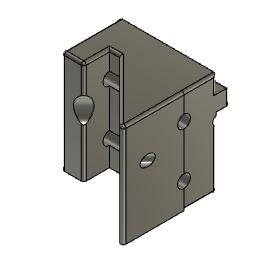
porte miroir ok v3 (Autodesk Fusion 360 design; units mm, degrees)
Autodesk Fusion 360 part; units mm, degrees
sketch "Sketch1" plane through (0, 0, 0) normal (0, 0, 1) x (1, 0, 0)
  line L0 (0, 0) -> (-12.5, 0)
  line L1 (-12.5, 0) -> (-12.5, -10)
  line L2 (0, 0) -> (25, -25)
  line L3 (0, 0) -> (25, 0)
  line L4 (25, 0) -> (25, -25)
  line L5 (-12.5, 0) -> (24.9893, 0)
  line L6 (24.9893, 0) -> (24.9893, 12.5)
  line L7 (24.9893, 12.5) -> (-12.5, 12.5)
  line L8 (-12.5, 12.5) -> (-12.5, 0)
  line L9 (-4, 0) -> (-4, -10)
  line L10 (-12.5, -10) -> (-4, -10)
  dimension "d27" = 12.5
  dimension "d28" = 12.5
  dimension "d29" = 10
  constraint coincident L0.start L2.start
  constraint horizontal L0
  constraint vertical L1
  constraint horizontal L5
  constraint vertical L6
  constraint horizontal L7
  constraint vertical L8
  constraint coincident L5 L9.start
  constraint perpendicular L9 L10
  measures "d27" distance of L0.start L0.end
  measures "d28" distance of L0.end L7.end
  measures "d29" distance of L0.end L1.end
extrude "Extrude7" add sketch "Sketch1" along normal blind 40
sketch "Sketch9" plane through (-12.5, 0, 0) normal (-1, 0, 0) x (0, -1, 0)
  line L0 (-12.5, 0) -> (10, 0)
  line L1 (10, 0) -> (10, 40)
  line L2 (10, 40) -> (-12.5, 40)
  line L3 (-12.5, 40) -> (-12.5, 0)
  circle A0 centre (0, 30) radius 2.5
  circle A1 centre (0, 10) radius 2.5
  dimension "d32" = 5
  dimension "d33" = 5
  dimension "d34" = 10
  dimension "d35" = 10
  dimension "d36" = 20
  measures "d32" diameter of A0
  measures "d33" diameter of A1
  measures "d34" distance of L2 A0.centre
  measures "d35" distance of L0 A1.centre
  measures "d36" distance of A0.centre A1.centre
extrude "Extrude8" cut sketch "Sketch9" against normal blind 50 contours A0 | A1
sketch "Sketch10" plane through (0, 0, 0) normal (-0.707107, -0.707107, 0) x (0.707107, -0.707107, 0)
  line L0 (0, 27.5) -> (0, 12.5)
  ellipse E0 centre (0, 10) end of major axis (3.5355, 10) minor radius 2.5 (0, 7.5) -> (0, 12.5) ccw
  line L1 (0, 7.5) -> (0, 0)
  line L2 (0, 0) -> (35.3553, 0)
  line L3 (35.3553, 0) -> (35.3553, 40)
  line L4 (35.3553, 40) -> (0, 40)
  line L5 (0, 40) -> (0, 32.5)
  ellipse E1 centre (0, 30) end of major axis (3.5355, 30) minor radius 2.5 (0, 27.5) -> (0, 32.5) ccw
  line L6 (17.6777, 24) -> (27.6777, 24)
  circle A0 centre (7.6777, 24) radius 2.1
  circle A1 centre (27.6777, 24) radius 2.1
  dimension "d41" = 4.2
  dimension "d42" = 4.2
  constraint coincident L6.end A1.centre
  measures "d41" diameter of A0
  measures "d42" diameter of A1
extrude "Extrude9" cut sketch "Sketch10" against normal blind 50 contours A0 | A1
sketch "Sketch11" plane through (0, 12.5, 0) normal (0, 1, 0) x (-1, 0, 0)
  ellipse E0 centre (-23.3579, 24) end of major axis (-26.3277, 24) minor radius 2.1 (-24.9893, 22.2452) -> (-24.9893, 25.7548) ccw
  line L0 (-24.9893, 22.2452) -> (-24.9893, 0)
  line L1 (-24.9893, 0) -> (12.5, 0)
  line L2 (12.5, 0) -> (12.5, 40)
  line L3 (12.5, 40) -> (-24.9893, 40)
  line L4 (-24.9893, 40) -> (-24.9893, 25.7548)
  circle A0 centre (-12.5453, 29.9363) radius 2.05
  dimension "d45" = 4.1
  measures "d45" diameter of A0
extrude "Extrude10" cut sketch "Sketch11" against normal blind 50 contours A0
ref_plane "WorkPlane1" through (6.2446, 7.5, 20) normal (0, 1, 0) x (-1, 0, 0)
sketch "Sketch12" plane through (6.2446, 7.5, 20) normal (0, 1, 0) x (1, 0, 0)
  circle A0 centre (6.3004, -9.9317) radius 4.1
  dimension "d49" = 8.2
  measures "d49" diameter of A0
extrude "Extrude11" cut sketch "Sketch12" against normal blind 50
move_face "OffsetFaces2" offset -2 1 faces at (11.1129, 7.5, 26.8414)
sketch "Sketch13" plane through (0, 12.5, 0) normal (0, 1, 0) x (-1, 0, 0)
  circle A0 centre (-12.5453, 29.9363) radius 2.05
  ellipse E0 centre (-23.3579, 24) end of major axis (-26.3277, 24) minor radius 2.1 (-24.9893, 22.2452) -> (-24.9893, 25.7548) ccw
  line L0 (-24.9893, 22.2452) -> (-24.9893, 0)
  line L1 (-24.9893, 0) -> (12.5, 0)
  line L2 (12.5, 0) -> (12.5, 40)
  line L3 (12.5, 40) -> (-24.9893, 40)
  line L4 (-24.9893, 40) -> (-24.9893, 25.7548)
  line L5 (-24.9893, 32.9363) -> (-24.9893, 26.9363)
  line L6 (-24.9893, 32.9363) -> (-18.9893, 32.9363)
  line L7 (-18.9893, 32.9363) -> (-18.9893, 26.9363)
  line L8 (-18.9893, 26.9363) -> (-24.9893, 26.9363)
  line L9 (-24.9893, 26.9363) -> (-24.9893, 32.9363)
  line L10 (12.5, 32.9363) -> (-6.2446, 32.9363)
  line L11 (-6.2446, 32.9363) -> (-6.2446, 26.9363)
  line L12 (-6.2446, 26.9363) -> (12.5, 26.9363)
  line L13 (12.5, 26.9363) -> (12.5, 32.9363)
  point P0 (-12.5453, 29.9363)
  dimension "d55" = 6
  constraint coincident P0 A0.centre
  constraint coincident L4 L5.start
  constraint coincident L4 L5.end
  constraint coincident L2 L10.start
  constraint horizontal L6
  constraint vertical L7
  constraint horizontal L8
  constraint vertical L9
  constraint horizontal L10
  constraint vertical L11
  constraint horizontal L12
  constraint vertical L13
  measures "d55" distance of L5.start L6.end
extrude "Extrude12" add sketch "Sketch13" along normal blind 5 contours L4 L5 L6 L7 L8 L9 | L2 L10 L11 L12 L13
fillet "Fillet1" radius 1 23 edges at (25, -25, 20) (-4, -10, 20) (-12.5, -10, 20) (24.9893, 12.5, 36.4681) (-12.5, 12.5, 36.4681) (-12.5, 1.25, 40) (-12.5, 1.25, 0) (6.2446, 12.5, 0) (25, -12.5, 40) (12.5, -12.5, 40) (-4, -5, 40) (-2, 0, 40) (-8.25, -10, 40) (24.9893, 6.25, 40) (-3.1277, 17.5, 32.9363) (-3.1277, 17.5, 26.9363) (6.2446, 17.5, 29.9363) (-12.5, 17.5, 29.9363) (18.9893, 17.5, 29.9363) (24.9893, 17.5, 29.9363) (21.9893, 17.5, 26.9363) (21.9893, 17.5, 32.9363) (-12.5, 12.5, 13.4681)
fillet "Fillet2" radius 1 3 edges at (24.9893, 5.75, 0) (24.9893, 12.2071, 0.2929) (24.9893, 12.5, 11.6226)
sketch "Sketch14" plane through (0, 0, 0) normal (-0.707107, -0.707107, 0) x (0.707107, -0.707107, 0)
  line L0 (32.9411, 0) -> (32.9411, 39)
  line L1 (32.9411, 39) -> (0, 39)
  line L2 (0, 39) -> (0, 32.5)
  ellipse E0 centre (0, 30) end of major axis (3.5355, 30) minor radius 2.5 (0, 27.5) -> (0, 32.5) ccw
  line L3 (0, 27.5) -> (0, 12.5)
  ellipse E1 centre (0, 10) end of major axis (3.5355, 10) minor radius 2.5 (0, 7.5) -> (0, 12.5) ccw
  line L4 (0, 7.5) -> (0, 0)
  line L5 (0, 0) -> (32.9411, 0)
  circle A0 centre (27.6777, 24) radius 2.1
  circle A1 centre (7.6777, 24) radius 2.1
  ellipse E2 centre (17.7414, 29.9317) end of major axis (23.5397, 29.9317) minor radius 4.1
  circle A2 centre (7.6777, 24) radius 6.25
  dimension "d60" = 12.5
  constraint concentric A1 A2
  measures "d60" diameter of A2
extrude "Extrude13" cut sketch "Sketch14" along normal blind 41 contours A2
